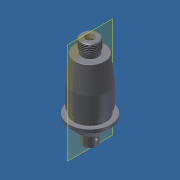
# Autodesk Inventor part: EIXO DA BETONEIRA(21)
Saved by Autodesk Inventor 2012 SP2 (Build 160219200, 219)
## iProperties
Created: 2012-07-23
Part Number: EIXO DA BETONEIRA(21)
Material: Carbon Steel
Document SubType Name: Modeling
Designer: bruno.silveira
Mass: 1384.32 g
Surface Area: 195.423 cm^2
Volume: 175.898 cm^3
Density: 7.87 g/cm^3
Author: bruno.silveira
Autodesk Inventor part; units mm, degrees
ref_plane "YZ Plane" through (0, 0, 0) normal (1, 0, 0) x (0, 1, 0)
ref_plane "XZ Plane" through (0, 0, 0) normal (0, 1, 0) x (-1, 0, 0)
ref_plane "XY Plane" through (0, 0, 0) normal (0, 0, 1) x (1, 0, 0)
sketch "Sketch1" plane through (0, 0, 0) normal (0, 0, 1) x (1, 0, 0)
  circle A0 centre (0, 0) radius 24.5
  dimension "d0" = 49
  constraints: 1 centre point, 1 coincident
  measures "d0" diameter of A0
extrude "Extrusion1" add sketch "Sketch1" along normal blind 110
sketch "Sketch2" plane through (0, 0, 110) normal (0, 0, 1) x (1, 0, 0)
  circle A0 centre (0, 0) radius 24.5 projected
  circle A1 centre (0, 0) radius 14
  dimension "d3" = 28
  constraints: 1 centre point, 1 coincident
  measures "d3" diameter of A1
extrude "Extrusion2" cut sketch "Sketch2" against normal blind 15
sketch "Sketch3" plane through (0, 0, 95) normal (0, 0, 1) x (1, 0, 0)
  circle A0 centre (0, 0) radius 24.5 projected
  circle A1 centre (0, 0) radius 22
  dimension "d6" = 44
  constraints: 1 centre point, 1 coincident
  measures "d6" diameter of A1
extrude "Extrusion3" cut sketch "Sketch3" against normal blind 60
sketch "Sketch4" plane through (0, 0, 0) normal (0, 0, -1) x (-1, 0, 0)
  circle A0 centre (0, 0) radius 24.5 projected
  circle A1 centre (0, 0) radius 10
  dimension "d9" = 20
  constraints: 1 centre point, 1 coincident
  measures "d9" diameter of A1
extrude "Extrusion4" cut sketch "Sketch4" against normal blind 17
chamfer "Chamfer1" distance 11 angle 45 1 edges at (-24.5, 0, 17) measured on face at (19.3325, 2.7521, 17)
sketch "Sketch5" plane through (0, 0, 95) normal (0, 0, 1) x (1, 0, 0)
  circle A0 centre (0, 0) radius 22 projected
  circle A1 centre (0, 0) radius 14 projected
extrude "Extrusion5" cut sketch "Sketch5" against normal blind 1
sketch "Sketch6" plane through (0, 0, 0) normal (0, 0, -1) x (-1, 0, 0)
  circle A0 centre (0, 0) radius 10 projected
extrude "Extrusion6" cut sketch "Sketch6" against normal blind 1
sketch "Sketch7" plane through (0, 0, 1) normal (0, 0, -1) x (-1, 0, 0)
  circle A0 centre (0, 0) radius 10 projected
  circle A1 centre (0, 0) radius 8
  dimension "d22" = 16
  constraints: 1 centre point, 1 coincident
  measures "d22" diameter of A1
extrude "Extrusion7" cut sketch "Sketch7" against normal blind 16
sketch "Sketch8" plane through (0, 0, 35) normal (0, 0, 1) x (1, 0, 0)
  circle A0 centre (0, 0) radius 22 projected
  circle A1 centre (0, 0) radius 24.5 projected
extrude "Extrusion8" cut sketch "Sketch8" against normal blind 3
sketch "Sketch9" plane through (0, 0, 0) normal (0, 1, 0) x (-1, 0, 0)
  line L0 (22, 32) -> (-22, 32) projected
  line L1 (-22, 40) -> (-19, 40)
  line L2 (-19, 40) -> (-19, 32)
  line L3 (-19, 32) -> (-22, 32)
  line L4 (-22, 32) -> (-22, 40)
  line L5 (0, 0) -> (0, 69)
  point P0 (22, 69)
  point P1 (-22, 69)
  dimension "d27" = 8
  dimension "d28" = 38
  dimension "d29" = 3
  constraints: 10 end point, 2 parallel, 1 horizontal, 1 perpendicular, 1 point on line
  measures "d27" distance of L3.end L1.start
  measures "d28" diameter of L2 L5
  measures "d29" distance between parallel lines of L2 L4
revolve "Revolution1" cut sketch "Sketch9" angle 360 about axis through (0, 0, 0) along (0, 0, 1)
sketch "Sketch11" plane through (0, 0, 94) normal (0, 0, 1) x (1, 0, 0)
  circle A0 centre (0, 0) radius 22 projected
  circle A1 centre (0, 0) radius 21
  dimension "d31" = 42
  constraints: 1 centre point, 1 coincident
  measures "d31" diameter of A1
extrude "Extrusion9" cut sketch "Sketch11" against normal blind 30
chamfer "Chamfer3" distance 30 angle 6 1 edges at (-21, 0, 94) measured on face at (20.7281, -3.3686, 74)
sketch "Sketch12" plane through (0, 0, 64) normal (0, 0, 1) x (1, 0, 0)
  circle A0 centre (0, 0) radius 21 projected
  circle A1 centre (0, 0) radius 22 projected
extrude "Extrusion10" cut sketch "Sketch12" against normal blind 28
sketch "Sketch13" plane through (0, 0, 110) normal (0, 0, 1) x (1, 0, 0)
  circle A0 centre (0, 0) radius 14 projected
  constraints: 1 coincident
hole "Hole1" at (0, 0, 110) direction (0, 0, -1) diameter 6.401 depth 35 tip angle 118 countersink diameter 10 countersink angle 60 thread size "5/16-18 UNC" class "2B" standard "ANSI Unified Screw Threads"
sketch "Sketch14" plane through (0, 0, 1) normal (0, 0, -1) x (-1, 0, 0)
  circle A0 centre (0, 0) radius 8 projected
  constraints: 1 coincident
hole "Hole2" at (0, 0, 1) direction (0, 0, 1) diameter 10 depth 32 tip angle 118 countersink diameter 11 countersink angle 60
sketch "Sketch16" plane through (0, 0, 110) normal (0, 0, 1) x (1, 0, 0)
  circle A0 centre (0, 0) radius 14 projected
  circle A1 centre (0, 0) radius 10.5
  dimension "d56" = 21
  constraints: 1 centre point, 1 coincident
  measures "d56" diameter of A1
extrude "Extrusion11" cut sketch "Sketch16" against normal blind 16
sketch "Sketch17" plane through (0, 0, 0) normal (1, 0, 0) x (0, 1, 0)
  line L0 (10.5, 94) -> (-10.5, 94) projected
  line L1 (10.5, 110) -> (-10.5, 110) projected
  line L2 (10.5, 94) -> (9.5, 94)
  line L3 (9.5, 94) -> (9.5, 100)
  line L4 (9.5, 100) -> (10.5, 100)
  line L5 (10.5, 100) -> (10.5, 94)
  line L6 (0, 110) -> (0, 0)
  dimension "d59" = 6
  dimension "d60" = 1
  constraints: 10 end point, 3 parallel, 1 horizontal, 1 midpoint, 1 perpendicular
  measures "d59" distance of L2.end L3.end
  measures "d60" distance between parallel lines of L5 L3
revolve "Revolution3" cut sketch "Sketch17" angle 360 about axis through (0, 0, 110) along (0, 0, -1)
thread "Thread1" size "7/8-14 UNF" class "2A" standard "ANSI Unified Screw Threads" full length
chamfer "Chamfer4" distance 1 angle 45 1 edges at (-10.5, 0, 110)
chamfer "Chamfer5" distance 0.5 angle 45 1 edges at (8, 0, 1)
fillet "Fillet1" radius 0.5 1 edges at (-17.8474, 0, 94)
sketch "Sketch18" plane through (0, 0, 0) normal (1, 0, 0) x (0, 1, 0)
  circle A0 centre (0, 9) radius 1.5
  line L0 (7.5, 1) -> (-7.5, 1) projected
  point P0 (0, 0)
  dimension "d71" = 3
  dimension "d72" = 8
  constraints: 1 centre point
  measures "d71" diameter of A0
  measures "d72" distance from line of L0 A0.centre
extrude "Extrusion12" cut sketch "Sketch18" along normal mid plane 25
body "Solid1"
